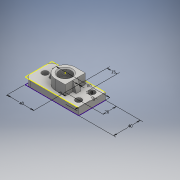
# Autodesk Inventor part: Основание1111
Saved by Autodesk Inventor 2016 (Build 200138000, 138)
## iProperties
Created: 2016-10-19
Part Number: Основание1111
Material: Типовые
Document SubType Name: Modeling
Designer: Student
Density: 1 g/cm^3
Appearance: По умолчанию
Mass: 37.0385 g
Surface Area: 119.555 cm^2
Volume: 37.0385 cm^3
Author: Student
Autodesk Inventor part; units mm, degrees
ref_plane "YZ Plane" through (0, 0, 0) normal (1, 0, 0) x (0, 1, 0)
ref_plane "XZ Plane" through (0, 0, 0) normal (0, 1, 0) x (-1, 0, 0)
ref_plane "XY Plane" through (0, 0, 0) normal (0, 0, 1) x (1, 0, 0)
sketch "Эскиз1" plane through (0, 0, 0) normal (0, 0, 1) x (1, 0, 0)
  line L0 (40, 20) -> (-40, 20)
  line L1 (-40, 20) -> (-40, -20)
  line L2 (-40, -20) -> (40, -20)
  line L3 (40, -20) -> (40, 20)
  line L4 (15, 15) -> (0, 15)
  line L5 (0, 15) -> (0, -15)
  line L6 (0, -15) -> (15, -15)
  line L7 (15, -15) -> (15, 15)
  arc A0 (0, 15) -> (0, -15) centre (0, 0) ccw
  point P0 (0, 0)
  dimension "d0" = 80
  dimension "d1" = 40
  dimension "d2" = 15
  dimension "d3" = 30
  dimension "d4" = 0
  dimension "d5" = 40
  dimension "d6" = 20
  dimension "d7" = 0
  constraints: 16 end point, 4 parallel, 2 horizontal, 2 perpendicular, 2 point on circle, 1 centre point, 1 midpoint
  measures "d0" distance of L0.start L0.end
  measures "d1" distance of L2.end L0.start
  measures "d2" distance of L4.start L4.end
  measures "d3" distance of L6.end L4.start
  measures "d4" distance of point (0, 0) A0.centre
  measures "d5" distance from line of point (0, 0) L1
  measures "d6" distance from line of point (0, 0) L0
  measures "d7" distance of point (0, 0) A0.centre
extrude "Выдавливание1" add sketch "Эскиз1" along normal blind 10
extrude "Выдавливание2" add sketch "Эскиз1" along normal blind 25 contours L7 L6 L5 L4 | L5 A0
ref_plane "РабПлоскость1" through (0, 0, 25) normal (0, 0, 1) x (1, 0, 0)
sketch "Эскиз2" plane through (0, 0, 25) normal (0, 0, 1) x (1, 0, 0)
  point P0 (0, 0)
  point P1 (0, 0)
  constraints: 1 coincident
hole "Отверстие1" at (0, 0, 25) direction (0, 0, -1) diameter 18.376 depth 20 thread size "M20x1.5" class "6H" standard "ANSI Metric M Profile"
chamfer "Фаска1" distance 1.6 angle 45 1 edges at (0, 9.188, 25)
ref_plane "РабПлоскость2" through (0, 0, 10) normal (0, 0, 1) x (1, 0, 0)
sketch "Эскиз3" plane through (0, 0, 10) normal (0, 0, 1) x (1, 0, 0)
  point P0 (0, 0)
  point P1 (-30, 0)
  point P2 (30, 10)
  point P3 (30, -10)
  dimension "d24" = 30
  dimension "d25" = 30
  dimension "d26" = 10
  dimension "d27" = 10
  dimension "d28" = 30
  measures "d24" distance of point (0, 0) point (-30, 0)
  measures "d25" horizontal distance of point (0, 0) point (30, 10)
  measures "d26" vertical distance of point (0, 0) point (30, 10)
  measures "d27" vertical distance of point (0, 0) point (30, -10)
  measures "d28" horizontal distance of point (0, 0) point (30, -10)
hole "Отверстие2" at (-30, 0, 10) at (30, 10, 10) at (30, -10, 10) direction (0, 0, -1) diameter 9 depth 20
ref_plane "РабПлоскость3" through (0, 0, 10) normal (0, -1, 0) x (1, 0, 0)
sketch "Эскиз4" plane through (0, 0, 10) normal (0, -1, 0) x (1, 0, 0)
  point P0 (0, -10)
sketch "Эскиз5" plane through (0, 0, 0) normal (0, 1, 0) x (-1, 0, 0)
  line L0 (-15, 10) -> (-15, 25) projected
  line L1 (-15, 25) -> (-20, 10)
  line L2 (-40, 10) -> (40, 10) projected
  point P0 (0, 0)
  dimension "d36" = 5
  constraints: 2 end point, 1 point on line
  measures "d36" distance from line of L0 L1.end
extrude "Ребро жесткости1" add sketch "Эскиз5" along normal mid plane 7 rib yes fills toward (-15.05, 17.5) open curves L0 L1
sketch "Эскиз6" plane through (0, 0, 25) normal (0, 0, 1) x (1, 0, 0)
  point P0 (0, 0)
sketch "Эскиз7" plane through (0, 0, 10) normal (0, 0, 1) x (1, 0, 0)
  line L0 (40, 20) -> (-40, 20) projected
  line L1 (-40, 20) -> (-40, -20) projected
  point P0 (0, 0)
fillet "Сопряжение1" radius 8 1 edges at (-40, -20, 5)
fillet "Сопряжение2" radius 8 1 edges at (-40, 20, 5)
sketch "Эскиз8" plane through (0, 0, 10) normal (0, -1, 0) x (1, 0, 0)
  line L0 (-15, 0) -> (-15, 15) projected
  line L1 (-15, 13.3302) -> (-20.9395, 0)
  point P0 (0, -10)
  constraints: 2 end point, 1 point on line
extrude "Ребро жесткости2" add sketch "Эскиз8" along normal mid plane 7 rib yes fills toward (-17.9241, 6.6448) open curves L1
sketch "Эскиз9" plane through (0, 0, 10) normal (0, 0, 1) x (1, 0, 0)
  line L0 (-40, -20) -> (40, -20) projected
  line L1 (-40, 20) -> (-40, -20) projected
  point P0 (0, 0)
sketch "Эскиз10" plane through (0, 0, 10) normal (0, 0, 1) x (1, 0, 0)
  point P0 (0, 0)
